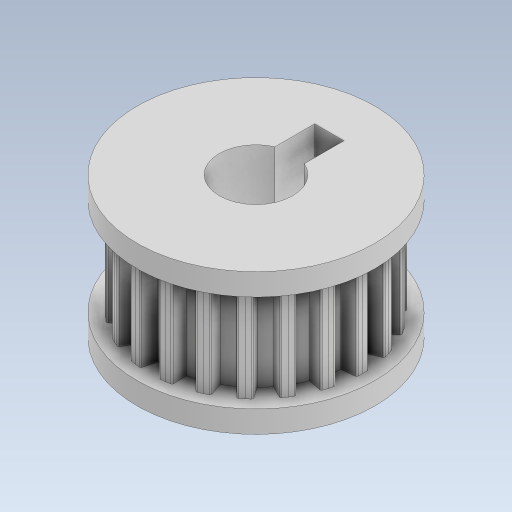
# Autodesk Inventor part: Rotor Pendorong
Saved by Autodesk Inventor 2023.5 (Build 275446000, 446)
## iProperties
Created: 2025-10-17
Part Number: Rotor Pendorong
Material: Generic
Document SubType Name: Modeling
Designer: Guntur
Density: 1 g/cm^3
Appearance: Default
Author: Guntur
## iProperties of the stored document Rotor Pendorong_3DPrint.ipt
Created: 2025-10-18
Part Number: Rotor Pendorong_3DPrint
Material: Generic
Document SubType Name: Modeling
Designer: Guntur
Density: 1 g/cm^3
Appearance: Default
Author: Guntur
Autodesk Inventor part; units mm, degrees
ref_plane "YZ Plane" through (0, 0, 0) normal (1, 0, 0) x (0, 1, 0)
ref_plane "XZ Plane" through (0, 0, 0) normal (0, 1, 0) x (-1, 0, 0)
ref_plane "XY Plane" through (0, 0, 0) normal (0, 0, 1) x (1, 0, 0)
sketch "Sketch1" plane through (0, 0, 0) normal (0, 1, 0) x (-1, 0, 0)
  circle A0 centre (0, 0) radius 2.5
  circle A1 centre (0, 0) radius 7.275
  circle A2 centre (0, 0) radius 7.275
  circle A3 centre (0, 0) radius 6.3
  line L0 (9.1935, 0) -> (-10, 0) construction
  line L1 (7.275, 0) -> (7.2664, 0.3121)
  line L2 (7.1766, 0.4088) -> (6.2801, 0.5005)
  arc A4 (7.2664, 0.3121) -> (7.1766, 0.4088) centre (7.1665, 0.3093) ccw
  line L3 (7.275, 0) -> (7.2664, -0.3121)
  line L4 (7.1766, -0.4088) -> (6.2801, -0.5005)
  arc A5 (7.1766, -0.4088) -> (7.2664, -0.3121) centre (7.1665, -0.3093) ccw
  point P0 (7.264, 0.3998)
  dimension "d3" = 12.6
  dimension "d0" = 5
  dimension "d2" = 14.55
  dimension "d4" = 0.4
  dimension "d5" = 0.1
  dimension "d26" = 14.55
  constraints: 10 end point, 6 point on circle, 5 centre point, 4 coincident, 4 symmetric about line, 3 point on line, 2 horizontal, 2 tangent, 4 other
  measures "d0" diameter of A0
  measures "d2" diameter of A2
  measures "d4" distance of L1.start A1.end
  measures "d5" radius of A4
  measures "d26" diameter of A1
extrude "Extrusion1" add sketch "Sketch1" along normal blind 6.6 contours A3
extrude "Extrusion2" add sketch "Sketch1" along normal blind 6.6 contours A1 A5 L4 A3 L2 A4 picked at (6.9162, 0.2266)
pattern_circular "Circular Pattern1" count 22 over 360 about axis through (0, 0, 0) along (0, 1, 0) of "Extrusion2"
sketch "Sketch2" plane through (0, 6.6, 0) normal (0, 1, 0) x (1, 0, 0)
  circle A0 centre (0, 0) radius 2.5
  circle A1 centre (0, 0) radius 8.1
  dimension "d13" = 16.2
  dimension "d22" = 5
  constraints: 2 centre point, 2 coincident
  measures "d13" diameter of A1
  measures "d22" diameter of A0
extrude "Extrusion3" add sketch "Sketch2" along normal blind 1.5
sketch "Sketch3" plane through (0, 0, 0) normal (0, -1, 0) x (1, 0, 0)
  circle A0 centre (0, 0) radius 2.5
  circle A1 centre (0, 0) radius 8.1
  arc A2 (-6.1667, 1.2891) -> (-6.2801, 0.5005) centre (0, 0) ccw projected
  line L0 (-7.1766, 0.4088) -> (-6.2801, 0.5005) projected
  arc A3 (-7.1766, 0.4088) -> (-7.2664, 0.3121) centre (-7.1665, 0.3093) ccw projected
  line L1 (-7.275, 0) -> (-7.2664, 0.3121) projected
  line L2 (-7.2664, -0.3121) -> (-7.275, 0) projected
  arc A4 (-7.2664, -0.3121) -> (-7.1766, -0.4088) centre (-7.1665, -0.3093) ccw projected
  line L3 (-6.2801, -0.5005) -> (-7.1766, -0.4088) projected
  arc A5 (-6.2801, -0.5005) -> (-6.1667, -1.2891) centre (0, 0) ccw projected
  line L4 (-7.0011, -1.6297) -> (-6.1667, -1.2891) projected
  arc A6 (-7.0011, -1.6297) -> (-7.06, -1.7478) centre (-6.9633, -1.7222) ccw projected
  line L5 (-6.9803, -2.0496) -> (-7.06, -1.7478) projected
  line L6 (-6.8842, -2.3466) -> (-6.9803, -2.0496) projected
  arc A7 (-6.8842, -2.3466) -> (-6.7708, -2.4141) centre (-6.789, -2.3158) ccw projected
  line L7 (-5.8847, -2.2495) -> (-6.7708, -2.4141) projected
  arc A8 (-5.8847, -2.2495) -> (-5.5537, -2.9742) centre (0, 0) ccw projected
  line L8 (-6.2584, -3.5361) -> (-5.5537, -2.9742) projected
  arc A9 (-6.2584, -3.5361) -> (-6.2816, -3.666) centre (-6.196, -3.6143) ccw projected
  line L9 (-6.1201, -3.9332) -> (-6.2816, -3.666) projected
  line L10 (-5.9442, -4.191) -> (-6.1201, -3.9332) projected
  arc A10 (-5.9442, -4.191) -> (-5.8164, -4.2239) centre (-5.8616, -4.1347) ccw projected
  line L11 (-5.0125, -3.8163) -> (-5.8164, -4.2239) projected
  arc A11 (-5.0125, -3.8163) -> (-4.4908, -4.4184) centre (0, 0) ccw projected
  line L12 (-5.0086, -5.156) -> (-4.4908, -4.4184) projected
  arc A12 (-5.0086, -5.156) -> (-4.9943, -5.2872) centre (-4.9268, -5.2135) ccw projected
  line L13 (-4.7641, -5.4981) -> (-4.9943, -5.2872) projected
  line L14 (-4.5227, -5.6959) -> (-4.7641, -5.4981) projected
  arc A13 (-4.5227, -5.6959) -> (-4.3908, -5.6914) centre (-4.4593, -5.6186) ccw projected
  line L15 (-3.7343, -5.0739) -> (-4.3908, -5.6914) projected
  arc A14 (-3.7343, -5.0739) -> (-3.0641, -5.5046) centre (0, 0) ccw projected
  line L16 (-3.3531, -6.3583) -> (-3.0641, -5.5046) projected
  arc A15 (-3.3531, -6.3583) -> (-3.3024, -6.4801) centre (-3.2584, -6.3903) ccw projected
  line L17 (-3.0221, -6.6176) -> (-3.3024, -6.4801) projected
  line L18 (-2.7347, -6.7394) -> (-3.0221, -6.6176) projected
  arc A16 (-2.7347, -6.7394) -> (-2.6094, -6.6979) centre (-2.6957, -6.6473) ccw projected
  line L19 (-2.1536, -5.9205) -> (-2.6094, -6.6979) projected
  arc A17 (-2.1536, -5.9205) -> (-1.3892, -6.1449) centre (0, 0) ccw projected
  line L20 (-1.426, -7.0454) -> (-1.3892, -6.1449) projected
  arc A18 (-1.426, -7.0454) -> (-1.343, -7.148) centre (-1.3261, -7.0495) ccw projected
  line L21 (-1.0353, -7.201) -> (-1.343, -7.148) projected
  line L22 (-0.7252, -7.2369) -> (-1.0353, -7.201) projected
  arc A19 (-0.7252, -7.2369) -> (-0.6167, -7.1618) centre (-0.7137, -7.1375) ccw projected
  line L23 (-0.3983, -6.2874) -> (-0.6167, -7.1618) projected
  arc A20 (-0.3983, -6.2874) -> (0.3983, -6.2874) centre (0, 0) ccw projected
  line L24 (0.6167, -7.1618) -> (0.3983, -6.2874) projected
  arc A21 (0.6167, -7.1618) -> (0.7252, -7.2369) centre (0.7137, -7.1375) ccw projected
  line L25 (1.0353, -7.201) -> (0.7252, -7.2369) projected
  line L26 (1.343, -7.148) -> (1.0353, -7.201) projected
  arc A22 (1.343, -7.148) -> (1.426, -7.0454) centre (1.3261, -7.0495) ccw projected
  line L27 (1.3892, -6.1449) -> (1.426, -7.0454) projected
  arc A23 (1.3892, -6.1449) -> (2.1536, -5.9205) centre (0, 0) ccw projected
  line L28 (2.6094, -6.6979) -> (2.1536, -5.9205) projected
  arc A24 (2.6094, -6.6979) -> (2.7347, -6.7394) centre (2.6957, -6.6473) ccw projected
  line L29 (3.0221, -6.6176) -> (2.7347, -6.7394) projected
  line L30 (3.3024, -6.4801) -> (3.0221, -6.6176) projected
  arc A25 (3.3024, -6.4801) -> (3.3531, -6.3583) centre (3.2584, -6.3903) ccw projected
  line L31 (3.0641, -5.5046) -> (3.3531, -6.3583) projected
  arc A26 (3.0641, -5.5046) -> (3.7343, -5.0739) centre (0, 0) ccw projected
  line L32 (4.3908, -5.6914) -> (3.7343, -5.0739) projected
  arc A27 (4.3908, -5.6914) -> (4.5227, -5.6959) centre (4.4593, -5.6186) ccw projected
  line L33 (4.7641, -5.4981) -> (4.5227, -5.6959) projected
  line L34 (4.9943, -5.2872) -> (4.7641, -5.4981) projected
  arc A28 (4.9943, -5.2872) -> (5.0086, -5.156) centre (4.9268, -5.2135) ccw projected
  line L35 (4.4908, -4.4184) -> (5.0086, -5.156) projected
  arc A29 (4.4908, -4.4184) -> (5.0125, -3.8163) centre (0, 0) ccw projected
  line L36 (5.8164, -4.2239) -> (5.0125, -3.8163) projected
  arc A30 (5.8164, -4.2239) -> (5.9442, -4.191) centre (5.8616, -4.1347) ccw projected
  line L37 (6.1201, -3.9332) -> (5.9442, -4.191) projected
  line L38 (6.2816, -3.666) -> (6.1201, -3.9332) projected
  arc A31 (6.2816, -3.666) -> (6.2584, -3.5361) centre (6.196, -3.6143) ccw projected
  line L39 (5.5537, -2.9742) -> (6.2584, -3.5361) projected
  arc A32 (5.5537, -2.9742) -> (5.8847, -2.2495) centre (0, 0) ccw projected
  line L40 (6.7708, -2.4141) -> (5.8847, -2.2495) projected
  arc A33 (6.7708, -2.4141) -> (6.8842, -2.3466) centre (6.789, -2.3158) ccw projected
  line L41 (6.9803, -2.0496) -> (6.8842, -2.3466) projected
  line L42 (7.06, -1.7478) -> (6.9803, -2.0496) projected
  arc A34 (7.06, -1.7478) -> (7.0011, -1.6297) centre (6.9633, -1.7222) ccw projected
  line L43 (6.1667, -1.2891) -> (7.0011, -1.6297) projected
  arc A35 (6.1667, -1.2891) -> (6.2801, -0.5005) centre (0, 0) ccw projected
  line L44 (7.1766, -0.4088) -> (6.2801, -0.5005) projected
  arc A36 (7.1766, -0.4088) -> (7.2664, -0.3121) centre (7.1665, -0.3093) ccw projected
  line L45 (7.275, 0) -> (7.2664, -0.3121) projected
  line L46 (7.2664, 0.3121) -> (7.275, 0) projected
  arc A37 (7.2664, 0.3121) -> (7.1766, 0.4088) centre (7.1665, 0.3093) ccw projected
  line L47 (6.2801, 0.5005) -> (7.1766, 0.4088) projected
  arc A38 (6.2801, 0.5005) -> (6.1667, 1.2891) centre (0, 0) ccw projected
  line L48 (7.0011, 1.6297) -> (6.1667, 1.2891) projected
  arc A39 (7.0011, 1.6297) -> (7.06, 1.7478) centre (6.9633, 1.7222) ccw projected
  line L49 (6.9803, 2.0496) -> (7.06, 1.7478) projected
  line L50 (6.8842, 2.3466) -> (6.9803, 2.0496) projected
  arc A40 (6.8842, 2.3466) -> (6.7708, 2.4141) centre (6.789, 2.3158) ccw projected
  line L51 (5.8847, 2.2495) -> (6.7708, 2.4141) projected
  arc A41 (5.8847, 2.2495) -> (5.5537, 2.9742) centre (0, 0) ccw projected
  line L52 (6.2584, 3.5361) -> (5.5537, 2.9742) projected
  arc A42 (6.2584, 3.5361) -> (6.2816, 3.666) centre (6.196, 3.6143) ccw projected
  line L53 (6.1201, 3.9332) -> (6.2816, 3.666) projected
  line L54 (5.9442, 4.191) -> (6.1201, 3.9332) projected
  arc A43 (5.9442, 4.191) -> (5.8164, 4.2239) centre (5.8616, 4.1347) ccw projected
  line L55 (5.0125, 3.8163) -> (5.8164, 4.2239) projected
  arc A44 (5.0125, 3.8163) -> (4.4908, 4.4184) centre (0, 0) ccw projected
  line L56 (5.0086, 5.156) -> (4.4908, 4.4184) projected
  arc A45 (5.0086, 5.156) -> (4.9943, 5.2872) centre (4.9268, 5.2135) ccw projected
  line L57 (4.7641, 5.4981) -> (4.9943, 5.2872) projected
  line L58 (4.5227, 5.6959) -> (4.7641, 5.4981) projected
  arc A46 (4.5227, 5.6959) -> (4.3908, 5.6914) centre (4.4593, 5.6186) ccw projected
  line L59 (3.7343, 5.0739) -> (4.3908, 5.6914) projected
  arc A47 (3.7343, 5.0739) -> (3.0641, 5.5046) centre (0, 0) ccw projected
  line L60 (3.3531, 6.3583) -> (3.0641, 5.5046) projected
  arc A48 (3.3531, 6.3583) -> (3.3024, 6.4801) centre (3.2584, 6.3903) ccw projected
  line L61 (3.0221, 6.6176) -> (3.3024, 6.4801) projected
  line L62 (2.7347, 6.7394) -> (3.0221, 6.6176) projected
  arc A49 (2.7347, 6.7394) -> (2.6094, 6.6979) centre (2.6957, 6.6473) ccw projected
  line L63 (2.1536, 5.9205) -> (2.6094, 6.6979) projected
  arc A50 (2.1536, 5.9205) -> (1.3892, 6.1449) centre (0, 0) ccw projected
  line L64 (1.426, 7.0454) -> (1.3892, 6.1449) projected
  arc A51 (1.426, 7.0454) -> (1.343, 7.148) centre (1.3261, 7.0495) ccw projected
  line L65 (1.0353, 7.201) -> (1.343, 7.148) projected
  line L66 (0.7252, 7.2369) -> (1.0353, 7.201) projected
  arc A52 (0.7252, 7.2369) -> (0.6167, 7.1618) centre (0.7137, 7.1375) ccw projected
  line L67 (0.3983, 6.2874) -> (0.6167, 7.1618) projected
  arc A53 (0.3983, 6.2874) -> (-0.3983, 6.2874) centre (0, 0) ccw projected
  line L68 (-0.6167, 7.1618) -> (-0.3983, 6.2874) projected
  arc A54 (-0.6167, 7.1618) -> (-0.7252, 7.2369) centre (-0.7137, 7.1375) ccw projected
  line L69 (-1.0353, 7.201) -> (-0.7252, 7.2369) projected
  line L70 (-1.343, 7.148) -> (-1.0353, 7.201) projected
  arc A55 (-1.343, 7.148) -> (-1.426, 7.0454) centre (-1.3261, 7.0495) ccw projected
  line L71 (-1.3892, 6.1449) -> (-1.426, 7.0454) projected
  arc A56 (-1.3892, 6.1449) -> (-2.1536, 5.9205) centre (0, 0) ccw projected
  line L72 (-2.6094, 6.6979) -> (-2.1536, 5.9205) projected
  arc A57 (-2.6094, 6.6979) -> (-2.7347, 6.7394) centre (-2.6957, 6.6473) ccw projected
  line L73 (-3.0221, 6.6176) -> (-2.7347, 6.7394) projected
  line L74 (-3.3024, 6.4801) -> (-3.0221, 6.6176) projected
  arc A58 (-3.3024, 6.4801) -> (-3.3531, 6.3583) centre (-3.2584, 6.3903) ccw projected
  line L75 (-3.0641, 5.5046) -> (-3.3531, 6.3583) projected
  arc A59 (-3.0641, 5.5046) -> (-3.7343, 5.0739) centre (0, 0) ccw projected
  line L76 (-4.3908, 5.6914) -> (-3.7343, 5.0739) projected
  arc A60 (-4.3908, 5.6914) -> (-4.5227, 5.6959) centre (-4.4593, 5.6186) ccw projected
  line L77 (-4.7641, 5.4981) -> (-4.5227, 5.6959) projected
  line L78 (-4.9943, 5.2872) -> (-4.7641, 5.4981) projected
  arc A61 (-4.9943, 5.2872) -> (-5.0086, 5.156) centre (-4.9268, 5.2135) ccw projected
  line L79 (-4.4908, 4.4184) -> (-5.0086, 5.156) projected
  arc A62 (-4.4908, 4.4184) -> (-5.0125, 3.8163) centre (0, 0) ccw projected
  line L80 (-5.8164, 4.2239) -> (-5.0125, 3.8163) projected
  arc A63 (-5.8164, 4.2239) -> (-5.9442, 4.191) centre (-5.8616, 4.1347) ccw projected
  line L81 (-6.1201, 3.9332) -> (-5.9442, 4.191) projected
  line L82 (-6.2816, 3.666) -> (-6.1201, 3.9332) projected
  arc A64 (-6.2816, 3.666) -> (-6.2584, 3.5361) centre (-6.196, 3.6143) ccw projected
  line L83 (-5.5537, 2.9742) -> (-6.2584, 3.5361) projected
  arc A65 (-5.5537, 2.9742) -> (-5.8847, 2.2495) centre (0, 0) ccw projected
  line L84 (-6.7708, 2.4141) -> (-5.8847, 2.2495) projected
  arc A66 (-6.7708, 2.4141) -> (-6.8842, 2.3466) centre (-6.789, 2.3158) ccw projected
  line L85 (-6.9803, 2.0496) -> (-6.8842, 2.3466) projected
  line L86 (-7.06, 1.7478) -> (-6.9803, 2.0496) projected
  arc A67 (-7.06, 1.7478) -> (-7.0011, 1.6297) centre (-6.9633, 1.7222) ccw projected
  line L87 (-6.1667, 1.2891) -> (-7.0011, 1.6297) projected
  circle A68 centre (0, 0) radius 2.5 projected
  dimension "d20" = 16.2
  dimension "d21" = 5
  constraints: 2 centre point, 2 coincident
  measures "d20" diameter of A1
  measures "d21" diameter of A0
extrude "Extrusion4" add sketch "Sketch3" along normal blind 1.5 contours A1 | L87 A67 L86 L85 A66 L84 A65 L83 A64 L82 L81 A63 L80 A62 L79 A61 L78 L77 A60 L76 A59 L75 A58 L74 L73 A57 L72 A56 L71 A55 L70 L69 A54 L68 A53 L67 A52 L66 L65 A51 L64 A50 L63 A49 L62 L61 A48 L60 A47 L59 A46 L58 L57 A45 L56 A44 L55 A43 L54 L53 A42 L52 A41 L51 A40 L50 L49 A39 L48 A38 L47 A37 L46 L45 A36 L44 A35 L43 A34 L42 L41 A33 L40 A32 L39 A31 L38 L37 A30 L36 A29 L35 A28 L34 L33 A27 L32 A26 L31 A25 L30 L29 A24 L28 A23 L27 A22 L26 L25 A21 L24 A20 L23 A19 L22 L21 A18 L20 A17 L19 A16 L18 L17 A15 L16 A14 L15 A13 L14 L13 A12 L12 A11 L11 A10 L10 L9 A9 L8 A8 L7 A7 L6 L5 A6 L4 A5 L3 A4 L2 L1 A3 L0 A2
sketch "Sketch5" plane through (0, -1.5, 0) normal (0, -1, 0) x (1, 0, 0)
  line L0 (1, -5) -> (-1, -5)
  line L1 (-1, -5) -> (-1, 0)
  line L2 (-1, 0) -> (1, 0)
  line L3 (1, 0) -> (1, -5)
  circle A0 centre (0, 0) radius 2.5 projected
  line L4 (1, -5) -> (-1, 0) construction
  line L5 (-1, -5) -> (1, 0) construction
  arc A1 (-2.1536, -5.9205) -> (-1.3892, -6.1449) centre (0, 0) ccw projected
  arc A2 (-2.1536, -5.9205) -> (-1.3892, -6.1449) centre (0, 0) ccw projected
  arc A3 (-0.3983, -6.2874) -> (0.3983, -6.2874) centre (0, 0) ccw projected
  arc A4 (-0.3983, -6.2874) -> (0.3983, -6.2874) centre (0, 0) ccw projected
  point P0 (0, -2.5)
  point P1 (1, -2.2913)
  point P2 (-1, -2.2913)
  dimension "d23" = 5
  constraints: 12 end point, 2 midpoint, 2 parallel, 1 horizontal, 1 perpendicular, 2 other
  measures "d23" distance of L0.end L1.end
extrude "Extrusion6" cut sketch "Sketch5" against normal blind 10 contours L0 L1 A0 L3
body "Solid1"
